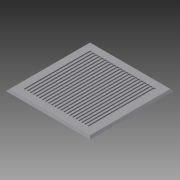
# Autodesk Inventor part: Element
Saved by Autodesk Inventor 2015 (Build 190159000, 159)
## iProperties
Created: 2016-03-23
Part Number: Element
Material: Generic
Document SubType Name: Modeling
Designer: Noah
Density: 1 g/cm^3
Appearance: Default
Author: Noah
Autodesk Inventor part; units mm, degrees
ref_plane "YZ Plane" through (0, 0, 0) normal (1, 0, 0) x (0, 1, 0)
ref_plane "XZ Plane" through (0, 0, 0) normal (0, 1, 0) x (-1, 0, 0)
ref_plane "XY Plane" through (0, 0, 0) normal (0, 0, 1) x (1, 0, 0)
sketch "Sketch1" plane through (0, 0, 0) normal (0, 0, 1) x (1, 0, 0)
  line L0 (-180, 180) -> (180, 180)
  line L1 (180, 180) -> (180, -180)
  line L2 (180, -180) -> (-180, -180)
  line L3 (-180, -180) -> (-180, 180)
  point P0 (0, 0)
  dimension "d0" = 360
  dimension "d1" = 360
  dimension "d2" = 180
  dimension "d3" = 180
  constraints: 8 end point, 2 parallel, 1 horizontal, 1 perpendicular
  measures "d0" distance of L0.start L0.end
  measures "d1" distance of L2.end L0.start
  measures "d2" distance from line of point (0, 0) L1
  measures "d3" distance from line of point (0, 0) L0
extrude "Extrusion1" add sketch "Sketch1" along normal blind 8
chamfer "Chamfer1" distance 8 angle 45 4 edges at (-180, 0, 8) (0, -180, 8) (180, 0, 8) (0, 180, 8)
sketch "Sketch3" plane through (0, 0, 8) normal (0, 0, 1) x (1, 0, 0)
  line L0 (-172, -172) -> (-172, 172) construction
  line L1 (-172, 142) -> (172, 142) construction
  line L2 (-172, 172) -> (172, 172) construction
  line L3 (-142, 172) -> (-142, -172) construction
  line L4 (172, -172) -> (-172, -172) construction
  line L5 (-172, -142) -> (172, -142) construction
  line L6 (172, 172) -> (172, -172) construction
  line L7 (142, 172) -> (142, -172) construction
  line L8 (-142, 142) -> (-132, 142)
  line L9 (-132, 142) -> (-132, -142)
  line L10 (-132, -142) -> (-142, -142)
  line L11 (-142, -142) -> (-142, 142)
  point P0 (0, 0)
  dimension "d12" = 30
  dimension "d13" = 30
  dimension "d14" = 30
  dimension "d15" = 30
  dimension "d16" = 10
  constraints: 16 end point, 10 point on line, 3 horizontal, 2 parallel, 2 perpendicular, 1 vertical
  measures "d12" distance between parallel lines of L3 L0
  measures "d13" distance between parallel lines of L1 L2
  measures "d14" distance between parallel lines of L4 L5
  measures "d15" distance between parallel lines of L7 L6
  measures "d16" distance of L9.end L10.end
extrude "Extrusion2" cut sketch "Sketch3" against normal blind 5
pattern_linear "Rectangular Pattern1" count 22 spacing 13 along (1, 0, 0) of "Extrusion2"
equation "\"d0\" = edge_length"
equation "\"d1\" = edge_length"
equation "\"d2\" = 0.5 * edge_length"
equation "\"d3\" = 0.5 * edge_length"
equation "\"d4\" = wall_width"
equation "\"d6\" = wall_width"
equation "\"d12\" = d13"
equation "\"d14\" = d13"
equation "\"d15\" = d13"
equation "\"edge_length\" = 360"
equation "\"wall_width\" = 8"
body "Solid1"
